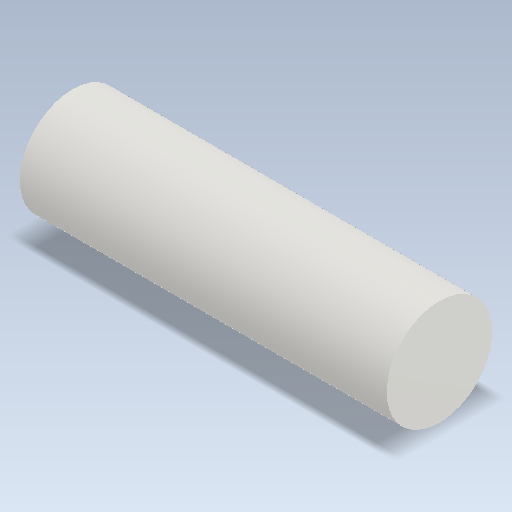
# Autodesk Inventor part: shaft_bar
Saved by Autodesk Inventor 2021 (Build 250183000, 183)
## iProperties
Created: 2023-08-21
Part Number: shaft_bar
Material: Acero inoxidable
Document SubType Name: Modeling
Designer: Sergio
Density: 8 g/cm^3
Appearance: Semipulido
Author: Sergio
Autodesk Inventor part; units mm, degrees
ref_plane "YZ Plane" through (0, 0, 0) normal (1, 0, 0) x (0, 1, 0)
ref_plane "XZ Plane" through (0, 0, 0) normal (0, 1, 0) x (-1, 0, 0)
ref_plane "XY Plane" through (0, 0, 0) normal (0, 0, 1) x (1, 0, 0)
sketch "Boceto1" plane through (0, 0, 0) normal (1, 0, 0) x (0, 1, 0)
  circle A0 centre (0, 0) radius 1.15
  dimension "d2" = 2.3
  constraints: 1 centre point, 1 coincident
  measures "d2" diameter of A0
extrude "Extrusión1" add sketch "Boceto1" along normal mid plane 8
equation "\"d2\" = wire_D"
equation "\"d0\" = width_link"
equation "\"thikness\" = 2"
equation "\"offset\" = 1"
equation "\"r1\" = 5.55"
equation "\"r2o\" = 59.75"
equation "\"delta_y\" = 6"
equation "\"wire_d\" = 1"
equation "\"width_ang_spring\" = 5"
equation "\"spring_int_diam\" = 8.5"
equation "\"spring_ext_diam\" = 10.5"
equation "\"r3\" = 8.25"
equation "\"r3R\" = 4.75"
equation "\"r3T\" = 6.74537"
equation "\"alpha\" = 54.847297deg"
equation "\"alpha2\" = 270deg"
equation "\"theta3_recogido\" = 305.152703deg"
equation "\"delta_theta_3\" = 45deg"
equation "\"joint_width\" = 12"
equation "\"joint_radius\" = 7.75"
equation "\"shaft_width\" = 15"
equation "\"shaft_joint_diameter\" = 7.75"
equation "\"separation_space\" = 0.5"
equation "\"height_finger\" = 42"
equation "\"cell_screw_head_diameter\" = 4"
equation "\"cell_screw_diameter\" = 2"
equation "\"cell_space\" = 2"
equation "\"cell_width\" = 6"
equation "\"cell_theta_position\" = 60deg"
equation "\"cell_thikness\" = 1"
equation "\"cell_lenght\" = 37"
equation "\"cell_z_space\" = 5"
equation "\"wire_D\" = 2.3"
equation "\"width_link\" = 8"
equation "\"Dt\" = 1.05949"
equation "\"Djoint_shaft\" = 2.3"
equation "\"shaft_x\" = 1.45"
equation "\"shaft_y\" = 6.45"
equation "\"lenght_body_link\" = 186.05"
equation "\"lenght_bar_support\" = 201.65"
equation "\"wire_spring_d\" = 1"
equation "\"spring_int_d\" = 6"
equation "\"spring_lenght\" = 28"
equation "\"trigger_offset\" = 2"
equation "\"m2_theta2o\" = 107deg"
equation "\"m2_r2\" = 28"
equation "\"e\" = 9"
equation "\"So\" = 17"
equation "\"m2_theta3o\" = -30deg"
equation "\"m2_r3\" = 19.75"
equation "\"m2_delta_theta1\" = 15deg"
equation "\"m2_theta3f\" = -60deg"
equation "\"trigger_thumb_lenght\" = 6"
equation "\"width_r12\" = 8"
equation "\"m2_r1\" = 25.2"
equation "\"r3_thikness\" = 3.5"
equation "\"t_thikness\" = 3"
equation "\"tg_width\" = 4"
equation "\"pivot_screw_d\" = 4"
equation "\"pivot_diameter\" = 7"
equation "\"sj_diam_shaft\" = 6"
equation "\"sj_groove\" = 2"
equation "\"sj_groove_deep\" = 7"
equation "\"sj_head_D\" = 7"
equation "\"sj_head_d\" = 4.7464"
equation "\"sj_head_height\" = 5"
equation "\"sf_lenght\" = 9.5"
equation "\"sf_base\" = 3"
equation "\"sf_head_height\" = 3"
equation "\"sf_head_width\" = 4.5"
equation "\"sf_head_offset\" = 0.25"
equation "\"sf_head_grip_width\" = 2"
equation "\"sf_head_angle\" = 45deg"
equation "\"sf_thikness\" = 5"
equation "\"screw_Dhead\" = 8"
equation "\"screw_d\" = 4"
equation "\"screw_lenght\" = 12"
equation "\"screwJ_base_D\" = 9"
equation "\"screwJ_top_D\" = 13"
equation "\"gj_D\" = 6"
equation "\"gj_d\" = 4"
equation "\"gj_out_section\" = 6"
equation "\"ext_width_slider\" = 3.5"
equation "\"sfbox_tip_width\" = 2.5"
equation "\"slim_width_slider\" = 1.5"
equation "\"agarradera_width\" = 4"
equation "\"int_width_slider\" = 2"
equation "\"agarradera_position\" = 82.13077"
equation "\"sfbox_theta1\" = 60deg"
equation "\"sfbox_theta2\" = 45deg"
equation "\"agarradera_theta\" = 60deg"
equation "\"sfbox_width\" = 1.5"
equation "\"box_fat_slider_lenght\" = 67"
equation "\"fat_width_slider\" = 2"
equation "\"box_in_width\" = 72"
equation "\"flex_separation_theta\" = 60deg"
equation "\"sf_flex_separation\" = 38.66667"
equation "\"thikness_box\" = 1.5"
equation "\"box_slim_slider_lenght\" = 116"
equation "\"box_in_deep\" = 77"
equation "\"box_in_height\" = 35"
